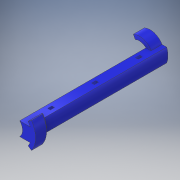
# Autodesk Inventor part: insert
Saved by Autodesk Inventor 2017 (Build 210142000, 142)
## iProperties
Created: 2018-12-03
Part Number: insert
Material: Generic
Document SubType Name: Modeling
Designer: ddeboer
Density: 1 g/cm^3
Appearance: Default
Author: ddeboer
Autodesk Inventor part; units mm, degrees
ref_plane "YZ Plane" through (0, 0, 0) normal (1, 0, 0) x (0, 1, 0)
ref_plane "XZ Plane" through (0, 0, 0) normal (0, 1, 0) x (-1, 0, 0)
ref_plane "XY Plane" through (0, 0, 0) normal (0, 0, 1) x (1, 0, 0)
sketch "Sketch1" plane through (0, 0, 0) normal (0, 0, 1) x (1, 0, 0)
  arc A0 (13.516009, -9.464011) -> (13.516009, 9.464011) centre (0, 0) ccw
  arc A1 (11.058553, -7.743282) -> (11.058553, 7.743282) centre (0, 0) ccw
  line L0 (11.058553, 7.743282) -> (13.516009, 9.464011)
  line L1 (0, 0) -> (16.5, 0) construction
  line L2 (11.058553, -7.743282) -> (13.516009, -9.464011)
  line L3 (0, 0) -> (16.5, 0) construction
  dimension "d0" = 33
  dimension "d1" = 27
  dimension "d2" = 35
  dimension "d3" = 35
  constraints: 8 end point, 4 point on circle, 2 centre point, 2 coincident, 2 horizontal
  measures "d0" diameter of A0
  measures "d1" diameter of A1
  measures "d2" angle of L1 L0
  measures "d3" angle of L2 L3
extrude "Extrusion1" add sketch "Sketch1" along normal blind 10
sketch "Sketch2" plane through (0, 0, 10) normal (0, 0, 1) x (1, 0, 0)
  line L0 (4.680418, -5.019579) -> (14.680418, -5.019579)
  line L1 (14.680418, -5.019579) -> (14.680418, 4.980421)
  line L2 (14.680418, 4.980421) -> (4.680418, 4.980421)
  line L3 (4.680418, 4.980421) -> (4.680418, -5.019579)
  line L4 (4.680418, -0.019579) -> (14.680418, -0.019579) construction
  point P0 (0, 0)
  dimension "d6" = 10
  dimension "d7" = 10
  constraints: 10 end point, 2 midpoint, 2 parallel, 1 horizontal, 1 perpendicular
  measures "d6" distance of L2.end L1.end
  measures "d7" distance of L1.end L0.end
extrude "Extrusion2" add sketch "Sketch2" against normal blind 100
sketch "Sketch4" plane through (0, 0, 0) normal (0, 0, -1) x (-1, 0, 0)
  circle A0 centre (0, 0) radius 18.238375
  circle A1 centre (0, 0) radius 13
  dimension "d14" = 26
  constraints: 2 centre point, 2 coincident
  measures "d14" diameter of A1
extrude "Extrusion4" cut sketch "Sketch4" along normal blind 100
sketch "Sketch5" plane through (0, 0, 10) normal (0, 0, 1) x (1, 0, 0)
  circle A0 centre (0, 0) radius 7
  dimension "d17" = 14
  constraints: 1 centre point, 1 coincident
  measures "d17" diameter of A0
extrude "Extrusion5" cut sketch "Sketch5" against normal blind 100
sketch "Sketch9" plane through (11.058553, 7.743282, 10) normal (-0.5735764, 0.819152, 0) x (0.819152, 0.5735764, 0)
  line L0 (-3.014035, 82) -> (-4.614035, 82)
  line L1 (-4.614035, 82) -> (-4.614035, 85)
  line L2 (-4.614035, 85) -> (-3.014035, 85)
  line L3 (-3.014035, 85) -> (-3.014035, 82)
  line L4 (-6.614035, 100) -> (-0.806856, 100)
  line L5 (-6.614035, 100) -> (-6.614035, 0)
  line L6 (-13.5, 120) -> (-13.5, -20)
  point P0 (-13.5, 10)
  dimension "d34" = 1.6
  dimension "d35" = 3
  dimension "d36" = 15
  dimension "d37" = 2
  constraints: 8 end point, 2 parallel, 1 horizontal, 1 perpendicular
  measures "d34" distance of L1.end L2.end
  measures "d35" distance of L0.end L1.end
  measures "d36" distance between parallel lines of L2 L4
  measures "d37" distance between parallel lines of L1 L5
revolve "Revolution4" cut sketch "Sketch9" angle 360 about axis through (0, 0, -10) along (0, 0, 1)
pattern_linear "Rectangular Pattern2" count 3 spacing 32 along (0, 0, 1) of "Revolution4"
ref_plane "Work Plane1" through (13.516009, -9.464011, 0) normal (-0.5735764, -0.819152, 0) x (0.819152, -0.5735764, 0)
sketch "Sketch10" plane through (13.516009, -9.464011, 0) normal (-0.5735764, -0.819152, 0) x (0.819152, -0.5735764, 0)
  line L0 (-15.327339, -90) -> (-9.52016, -90)
  line L1 (-9.52016, -90) -> (-6.52016, -90)
  line L2 (-6.52016, -90) -> (-6.52016, -82)
  line L3 (-6.52016, -82) -> (-9.52016, -82)
  line L4 (-9.52016, -82) -> (-9.52016, -90)
  line L5 (-16.5, -110) -> (-16.5, 30)
  point P0 (-16.5, 0)
  dimension "d43" = 3
  dimension "d44" = 8
  constraints: 8 end point, 2 parallel, 1 horizontal, 1 perpendicular
  measures "d43" distance of L3.end L2.end
  measures "d44" distance of L2.end L1.end
revolve "Revolution5" add sketch "Sketch10" angle 360 about axis through (0, 0, -10) along (0, 0, 1)
sketch "Sketch12" plane through (0, 0, -90) normal (0, 0, -1) x (-1, 0, 0)
  line L0 (0, 0) -> (9.97984, 0) construction
  arc A0 (-4.918883, 4.980421) -> (-4.878916, -5.019579) centre (0, 0) ccw
  line L1 (0, 0) -> (9.97984, 0) construction
  line L2 (0, 0) -> (5.071419, 10.875693)
  line L3 (0, 0) -> (12, 0) construction
  line L4 (0, 0) -> (5.494037, -11.782001)
  line L5 (0, 0) -> (13, 0) construction
  arc A1 (5.071419, -10.875693) -> (5.071419, 10.875693) centre (0, 0) ccw
  dimension "d53" = 65
  dimension "d54" = 65
  dimension "d56" = 13
  dimension "d57" = 12
  constraints: 12 end point, 4 horizontal, 2 equal length, 2 point on circle, 1 centre point, 1 coincident, 1 point on line
  measures "d53" angle of L3 L2
  measures "d54" angle of L4 L5
  measures "d56" distance of L1.start L4.end
  measures "d57" distance of L1.start L2.end
extrude "Extrusion8" cut sketch "Sketch12" against normal blind 10
chamfer "Chamfer2" distance 2 angle 45 1 edges at (16.5, 0, 0)
chamfer "Chamfer3" distance 1 angle 45 1 edges at (14.5, 0, 0)
body "Solid1"
